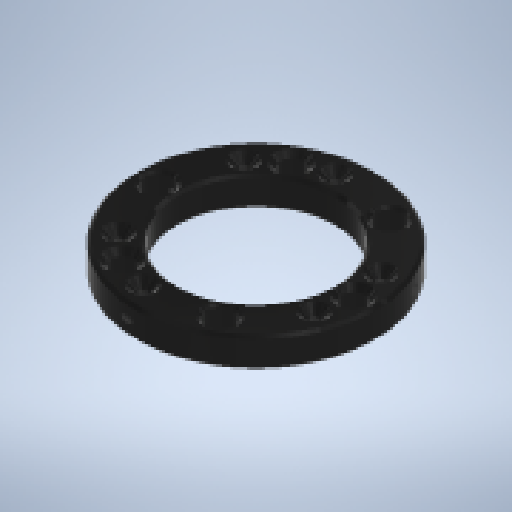
# Autodesk Inventor part: anneau
Saved by Autodesk Inventor 2024.2 (Build 282272000, 272)
## iProperties
Created: 2024-09-15
Part Number: anneau
Material: Générique
Document SubType Name: Modeling
Designer: Sebastien
Density: 1 g/cm^3
Appearance: Lisse - Noir
Author: Sebastien
Autodesk Inventor part; units mm, degrees
ref_plane "YZ Plane" through (0, 0, 0) normal (1, 0, 0) x (0, 1, 0)
ref_plane "XZ Plane" through (0, 0, 0) normal (0, 1, 0) x (-1, 0, 0)
ref_plane "XY Plane" through (0, 0, 0) normal (0, 0, 1) x (1, 0, 0)
sketch "Esquisse1" plane through (0, 0, 0) normal (0, 1, 0) x (-1, 0, 0)
  circle A0 centre (0, 0) radius 44.1
  circle A1 centre (36, 0) radius 5.15
  circle A2 centre (-18, 31.1769) radius 5.15
  circle A3 centre (-18, -31.1769) radius 5.15
  circle A4 centre (0, 0) radius 29
  circle A5 centre (-36, 0) radius 4.25
  circle A6 centre (18, -31.1769) radius 4.25
  circle A7 centre (18, 31.1769) radius 4.25
  arc A8 (6.2513, -35.4531) -> (27.5776, -23.1404) centre (0, 0) ccw construction
  point P0 (27.5776, 23.1404)
  point P1 (6.2513, 35.4531)
  point P2 (-33.8289, 12.3127)
  point P3 (-33.8289, -12.3127)
  point P4 (18, -31.1769)
  dimension "d0" = 88.2
  dimension "d1" = 10.3
  dimension "d2" = 36
  dimension "d5" = 360
  dimension "d9" = 58
  dimension "d13" = 8.5
  dimension "d14" = 36
  dimension "d17" = 360
  dimension "d32" = 40
  dimension "d35" = 360
  constraints: 9 centre point, 5 coincident, 3 point on circle, 2 horizontal alignment, 21 other
  measures "d0" diameter of A0
  measures "d1" diameter of A1
  measures "d2" distance of point (0, 0) A1.centre
  measures "d9" diameter of A4
  measures "d13" diameter of A5
  measures "d14" distance of point (0, 0) A5.centre
extrude "Extrusion1" add sketch "Esquisse1" against normal blind 11
chamfer "Chanfrein1" distance 1 angle 45 10 edges at (44.1, -11, 0) (29, -11, 0) (29, 0, 0) (44.1, 0, 0) (-30.85, 0, 0) (-30.85, -11, 0) (23.15, 0, -31.1769) (23.15, -11, -31.1769) (23.15, -11, 31.1769) (23.15, 0, 31.1769)
chamfer "Chanfrein2" distance 2 angle 45 6 edges at (40.25, -11, 0) (-13.75, -11, -31.1769) (-13.75, -11, 31.1769) (-13.75, 0, 31.1769) (-13.75, 0, -31.1769) (40.25, 0, 0)
sketch "Esquisse2" plane through (0, 0, 0) normal (0, 0, 1) x (1, 0, 0)
  line L0 (-36, -10) -> (-36, -1) construction
  line L1 (-41.15, -1) -> (-30.85, -1) construction
  line L2 (-30.85, -10) -> (-41.15, -10) construction
  point P0 (0, 0)
  point P1 (-31, -5)
  point P2 (-41, -5)
  point P3 (-36, -5.5)
  point P4 (-36, -5.5)
  constraints: 3 midpoint, 2 end point, 1 coincident, 1 vertical
hole "Perçage1" at (-36, -5.5, 0) direction (0, 0, -1) diameter 2.459 end through all thread size "M3x0.5" class "6H" standard "ISO Metric profile"
pattern_circular "Réseau circulaire1" count 3 over 360 about axis through (0, -10, 0) along (0, 1, 0) of "Perçage1"
hole "Perçage2" at (-6.2513, 0, -35.4531) at (-27.5776, 0, -23.1404) at (-27.5776, 0, 23.1404) at (-6.2513, 0, 35.4531) at (33.8289, 0, 12.3127) at (33.8289, 0, -12.3127) direction (0, -1, 0) diameter 3.242 end through all countersink diameter 9.4 countersink angle 90 thread size "M4x0.7" class "6H" standard "ISO Metric profile"
equation "\"d14\" = d2"
